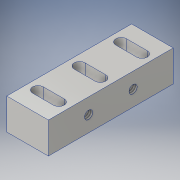
# Autodesk Inventor part: Motor Base
Saved by Autodesk Inventor 2016 (Build 200138000, 138)
## iProperties
Created: 2015-06-04
Part Number: Motor Base
Material: Aluminum 6061
Document SubType Name: Modeling
Designer: Dennis
Density: 2.7 g/cm^3
Appearance: Aluminum - Flat
Author: Dennis
Autodesk Inventor part; units mm, degrees
ref_plane "YZ Plane" through (0, 0, 0) normal (1, 0, 0) x (0, 1, 0)
ref_plane "XZ Plane" through (0, 0, 0) normal (0, 1, 0) x (-1, 0, 0)
ref_plane "XY Plane" through (0, 0, 0) normal (0, 0, 1) x (1, 0, 0)
sketch "Sketch1" plane through (0, 0, 0) normal (0, 0, 1) x (1, 0, 0)
  line L0 (0, 0) -> (25.4, 0)
  line L1 (25.4, 0) -> (25.4, 19.05)
  line L2 (25.4, 19.05) -> (0, 19.05)
  line L3 (0, 19.05) -> (0, 0)
  dimension "d0" = 25.4
  dimension "d1" = 19.05
  constraints: 8 end point, 2 parallel, 1 horizontal, 1 perpendicular
  measures "d0" distance of L0.start L0.end
  measures "d1" distance of L2.end L0.start
extrude "Extrusion1" add sketch "Sketch1" along normal blind 76.2
sketch "Sketch2" plane through (25.4, 0, 0) normal (1, 0, 0) x (0, 0, -1)
  line L0 (0, 0) -> (0, 19.05) projected
  line L1 (0, 19.05) -> (-76.2, 19.05) projected
  point P0 (-51.6636, 9.525)
  point P1 (-24.5364, 9.525)
  dimension "d4" = 27.1272
  dimension "d6" = 9.525
  dimension "d7" = 9.525
  dimension "d29" = 24.5364
  measures "d4" distance of point (-24.536, 9.525) point (-51.664, 9.525)
  measures "d6" distance from line of point (-24.536, 9.525) L1
  measures "d7" distance from line of point (-51.664, 9.525) L1
  measures "d29" distance from line of point (-24.536, 9.525) L0
hole "Hole1" at (25.4, 9.525, 51.6636) at (25.4, 9.525, 24.5364) direction (-1, 0, 0) diameter 4.9784 depth 22.225 tip angle 118 thread size "1/4-20 UNC" class "2B" standard "ANSI Unified Screw Threads"
sketch "Sketch3" plane through (0, 19.05, 0) normal (0, 1, 0) x (1, 0, 0)
  line L0 (6.35, -12.7) -> (19.05, -12.7) construction
  line L1 (6.35, -16.002) -> (19.05, -16.002)
  line L2 (19.05, -9.398) -> (6.35, -9.398)
  arc A0 (6.35, -9.398) -> (6.35, -16.002) centre (6.35, -12.7) ccw
  arc A1 (19.05, -16.002) -> (19.05, -9.398) centre (19.05, -12.7) ccw
  line L3 (6.35, -63.5) -> (19.05, -63.5) construction
  line L4 (6.35, -66.802) -> (19.05, -66.802)
  line L5 (19.05, -60.198) -> (6.35, -60.198)
  arc A2 (6.35, -60.198) -> (6.35, -66.802) centre (6.35, -63.5) ccw
  arc A3 (19.05, -66.802) -> (19.05, -60.198) centre (19.05, -63.5) ccw
  line L6 (6.35, -38.1) -> (19.05, -38.1) construction
  line L7 (6.35, -41.402) -> (19.05, -41.402)
  line L8 (19.05, -34.798) -> (6.35, -34.798)
  arc A4 (6.35, -34.798) -> (6.35, -41.402) centre (6.35, -38.1) ccw
  arc A5 (19.05, -41.402) -> (19.05, -34.798) centre (19.05, -38.1) ccw
  line L9 (25.4, 0) -> (25.4, -76.2) projected
  line L10 (25.4, -76.2) -> (0, -76.2) projected
  point P0 (12.7, -12.7)
  point P1 (12.7, -63.5)
  point P2 (12.7, -38.1)
  dimension "d15" = 3.302
  dimension "d16" = 3.302
  dimension "d17" = 3.302
  dimension "d18" = 12.7
  dimension "d19" = 12.7
  dimension "d20" = 12.7
  dimension "d21" = 25.4
  dimension "d22" = 25.4
  dimension "d23" = 6.35
  dimension "d24" = 6.35
  dimension "d25" = 6.35
  dimension "d26" = 12.7
  constraints: 24 end point, 12 point on circle, 12 tangent, 6 centre point, 4 parallel, 3 midpoint, 2 horizontal
  measures "d15" radius of A1
  measures "d16" radius of A5
  measures "d17" radius of A3
  measures "d18" distance of L0.start L0.end
  measures "d19" distance of L6.start L6.end
  measures "d20" distance of L3.start L3.end
  measures "d21" distance of point (12.7, -38.1) point (12.7, -12.7)
  measures "d22" distance of point (12.7, -63.5) point (12.7, -38.1)
  measures "d23" distance from line of L3.end L9
  measures "d24" distance from line of L6.end L9
  measures "d25" distance from line of L0.end L9
  measures "d26" distance from line of point (12.7, -63.5) L10
extrude "Extrusion2" cut sketch "Sketch3" against normal blind 101.6
body "Solid1"
